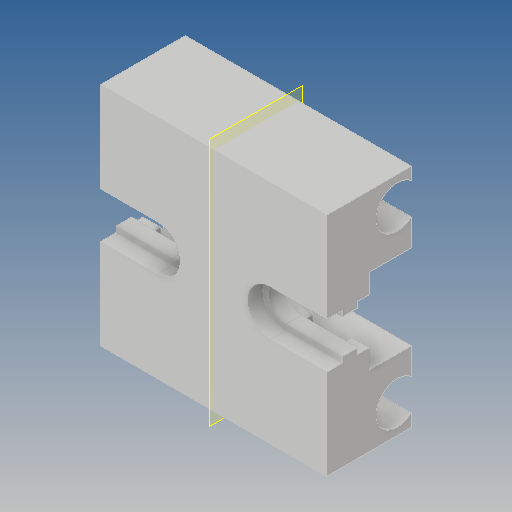
# Autodesk Inventor part: HotendMountCarriage
Saved by Autodesk Inventor 2018 (Build 220112000, 112)
## iProperties
Created: 2022-08-29
Part Number: HotendMountCarriage
Material: Generic
Document SubType Name: Modeling
Designer: Nathann
Density: 1 g/cm^3
Appearance: Default
Author: Nathann
Autodesk Inventor part; units mm, degrees
ref_plane "YZ Plane" through (0, 0, 0) normal (1, 0, 0) x (0, 1, 0)
ref_plane "XZ Plane" through (0, 0, 0) normal (0, 1, 0) x (-1, 0, 0)
ref_plane "XY Plane" through (0, 0, 0) normal (0, 0, 1) x (1, 0, 0)
sketch "Sketch1" plane through (0, 0, 0) normal (0, 0, 1) x (1, 0, 0)
  line L0 (0, 0) -> (80, 0)
  line L1 (80, 0) -> (80, -80)
  line L2 (80, -80) -> (0, -80)
  line L3 (0, -80) -> (0, 0)
  dimension "d0" = 80
  dimension "d1" = 80
  constraints: 8 end point, 2 parallel, 1 horizontal, 1 perpendicular
  measures "d0" distance of L0.start L0.end
  measures "d1" distance of L2.end L0.start
extrude "Extrusion1" add sketch "Sketch1" along normal blind 15
sketch "Sketch2" plane through (0, 0, 0) normal (0, 0, -1) x (-1, 0, 0)
  line L0 (0, 0) -> (-80, 0) projected
  circle A0 centre (-60, -40) radius 6.1
  line L1 (-80, 0) -> (-80, -80) projected
  line L2 (-60, -33.9) -> (-80, -33.9)
  line L3 (-80, -80) -> (-80, 0) projected
  line L4 (-60, -46.1) -> (-80, -46.1)
  line L5 (-80, -46.1) -> (-80, -33.9)
  dimension "d7" = 40
  dimension "d8" = 20
  dimension "d9" = 12.2
  constraints: 6 end point, 2 perpendicular, 2 point on circle, 2 point on line, 1 centre point, 1 horizontal
  measures "d7" distance from line of L0 A0.centre
  measures "d8" distance from line of L1 A0.centre
  measures "d9" diameter of A0
extrude "Extrusion2" cut sketch "Sketch2" against normal through all
sketch "Sketch3" plane through (0, 0, 0) normal (0, 0, -1) x (-1, 0, 0)
  arc A0 (-60, -46.1) -> (-60, -33.9) centre (-60, -40) ccw projected
  circle A1 centre (-60, -40) radius 8.1
  line L0 (-60, -31.9) -> (-80, -31.9)
  line L1 (-80, -33.9) -> (-80, 0) projected
  line L2 (-60, -48.1) -> (-80, -48.1)
  line L3 (-80, -48.1) -> (-80, -31.9)
  point P0 (0, 0)
  dimension "d12" = 16.2
  constraints: 6 end point, 2 horizontal, 2 point on circle, 1 centre point, 1 coincident, 1 perpendicular, 1 point on line
  measures "d12" diameter of A1
extrude "Extrusion3" cut sketch "Sketch3" against normal blind 4
sketch "Sketch4" plane through (0, 0, 15) normal (0, 0, 1) x (1, 0, 0)
  line L0 (80, -31.9) -> (60, -31.9) projected
  arc A0 (60, -31.9) -> (60, -48.1) centre (60, -40) ccw projected
  line L1 (60, -48.1) -> (80, -48.1) projected
  line L2 (80, -46.1) -> (60, -46.1) projected
  arc A1 (60, -33.9) -> (60, -46.1) centre (60, -40) ccw projected
  line L3 (60, -33.9) -> (80, -33.9) projected
  line L4 (80, -33.9) -> (80, -31.9)
  line L5 (80, -33.9) -> (80, 0) projected
  line L6 (80, -46.1) -> (80, -48.1)
  line L7 (80, -80) -> (80, -46.1) projected
  point P0 (0, 0)
  constraints: 4 end point, 2 collinear
extrude "Extrusion4" cut sketch "Sketch4" against normal blind 5.5
sketch "Sketch5" plane through (0, 0, 0) normal (0, 0, -1) x (-1, 0, 0)
  arc A0 (-60, -46.1) -> (-60, -33.9) centre (-60, -40) ccw projected
  line L0 (-80, -31.9) -> (-60, -31.9) projected
  circle A1 centre (-60, -40) radius 8.1
  line L1 (-60, -31.9) -> (-60, -31.9)
  line L2 (-73.8, -31.9) -> (-73.8, -48.1)
  line L3 (-60, -48.1) -> (-60, -48.1)
  arc A2 (-60, -48.1) -> (-60, -31.9) centre (-60, -40) ccw projected
  line L4 (-60, -31.9) -> (-60, -31.9)
  line L5 (-60, -31.9) -> (-60, -31.9)
  line L6 (-60, -33.9) -> (-60, -46.1)
  arc A3 (-60, -31.9) -> (-73.8, -31.9) centre (-66.9, -31.9) ccw
  arc A4 (-73.8, -48.1) -> (-60, -48.1) centre (-66.9, -48.1) ccw
  point P0 (0, 0)
  dimension "d17" = 13.8
  dimension "d20" = 16.2
  dimension "d21" = 8.1
  dimension "d37" = 0
  constraints: 12 end point, 7 point on circle, 5 vertical, 4 tangent, 3 centre point, 1 coincident, 1 parallel
  measures "d17" distance of L1.end L2.start
  measures "d20" distance of A4.centre A3.centre
  measures "d21" vertical distance of A1.centre A3.centre
  measures "d37" distance of L0.end L1.end
extrude "Extrusion5" cut sketch "Sketch5" against normal blind 4 contours A3 L0 | L0 A1 A4 L2
sketch "Sketch6" plane through (80, 0, 15) normal (1, 0, 0) x (0, 0, -1)
  line L0 (15, 0) -> (0, 0) projected
  line L1 (15, 0) -> (30, 0)
  line L2 (30, -25) -> (15, -25)
  line L3 (15, -25) -> (15, 0)
  line L4 (15, -80) -> (0, -80) projected
  line L5 (15, -80) -> (30, -80)
  line L6 (30, -55) -> (15, -55)
  line L7 (15, -55) -> (15, -80)
  arc A0 (30, -4.4098) -> (30, -15.5902) centre (25, -10) ccw
  arc A1 (30, -64.4098) -> (30, -75.5902) centre (25, -70) ccw
  line L8 (30, 0) -> (30, -4.4098)
  line L9 (30, -15.5902) -> (30, -25)
  line L10 (30, -80) -> (30, -75.5902)
  line L11 (30, -64.4098) -> (30, -55)
  dimension "d22" = 25
  dimension "d23" = 25
  dimension "d24" = 15
  dimension "d25" = 15
  dimension "d29" = 15
  dimension "d32" = 15
  dimension "d33" = 5
  dimension "d34" = 5
  dimension "d38" = 15
  dimension "d39" = 15
  dimension "d40" = 60
  dimension "d41" = 10
  dimension "d42" = 10
  constraints: 20 end point, 6 parallel, 4 perpendicular, 4 point on circle, 2 centre point, 2 horizontal
  measures "d22" distance of L1.end L2.start
  measures "d23" distance of L5.end L6.start
  measures "d24" distance of L4.start L5.end
  measures "d25" distance of L0.start L1.end
  measures "d29" diameter of A0
  measures "d32" diameter of A1
  measures "d33" distance from line of L8 A0.centre
  measures "d34" distance from line of A1.centre L11
  measures "d38" distance of L2.start L2.end
  measures "d39" distance of L6.start L6.end
  measures "d40" distance of A0.centre A1.centre
  measures "d41" distance from line of L5 A1.centre
  measures "d42" distance from line of L1 A0.centre
extrude "Extrusion6" add sketch "Sketch6" against normal blind 80
ref_plane "Work Plane1" through (40, -33.9, 4) normal (1, 0, 0) x (0, 0, -1)
mirror "Mirror1" about plane through (40, -33.9, 4) normal (1, 0, 0) of "Extrusion5", "Extrusion4", "Extrusion3", "Extrusion2"
equation "\"d24\" = d25"
equation "\"d32\" = d29"
equation "\"d34\" = d33"
equation "\"RodDiameter\" = 8"
equation "\"VerticalBearingOD\" = 16"
equation "\"PrintingClearance\" = 0.2"
equation "\"d31\" = d30"
equation "\"d30\" = 5"
body "Solid1"
